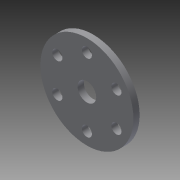
# Autodesk Inventor part: Hub for rachet
Saved by Autodesk Inventor 2013 (Build 170138000, 138)
## iProperties
Created: 2013-02-04
Part Number: Hub for rachet
Material: Generic
Document SubType Name: Modeling
Designer: Arpan
Density: 1 g/cm^3
Author: Arpan
Autodesk Inventor part; units mm, degrees
ref_plane "YZ Plane" through (0, 0, 0) normal (1, 0, 0) x (0, 1, 0)
ref_plane "XZ Plane" through (0, 0, 0) normal (0, 1, 0) x (-1, 0, 0)
ref_plane "XY Plane" through (0, 0, 0) normal (0, 0, 1) x (1, 0, 0)
sketch "Sketch1" plane through (0, 0, 0) normal (0, 0, 1) x (1, 0, 0)
  circle A0 centre (0, 0) radius 4.7625
  circle A1 centre (0, 0) radius 23.8125
  line L0 (0, 4.7625) -> (0, 17.4625)
  circle A2 centre (0, 17.4625) radius 2.5908
  circle A3 centre (-15.123, 8.7313) radius 2.5908
  circle A4 centre (-15.123, -8.7312) radius 2.5908
  circle A5 centre (0, -17.4625) radius 2.5908
  circle A6 centre (15.123, -8.7313) radius 2.5908
  circle A7 centre (15.123, 8.7312) radius 2.5908
  dimension "d0" = 9.525
  dimension "d1" = 47.625
  dimension "d2" = 12.7
  dimension "d3" = 5.1816
  dimension "d6" = 360
  constraints: 7 centre point, 3 coincident, 2 end point, 1 vertical, 1 vertical alignment, 15 other
  measures "d1" diameter of A1
  measures "d2" distance of L0.start L0.end
  measures "d3" diameter of A2
extrude "Extrusion1" add sketch "Sketch1" along normal blind 3.175
body "Solid1"
